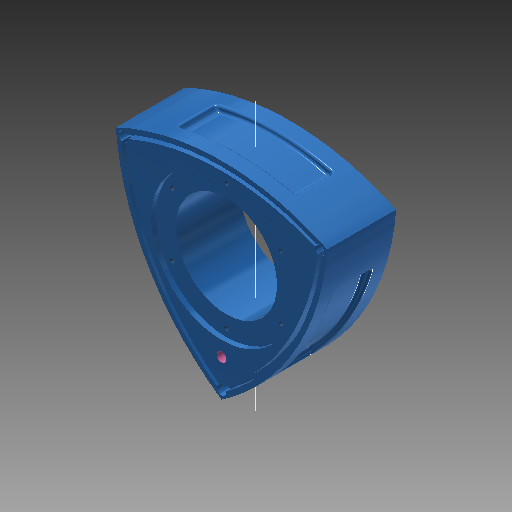
# Autodesk Inventor part: Rotor
Saved by Autodesk Inventor 2019.4 (Build 234330000, 330)
## iProperties
Created: 2020-05-01
Part Number: Rotor
Document SubType Name: Modeling
Designer: Gabriel
Material: Generic
Density: 1 g/cm^3
Appearance: Cyan
Author: Gabriel
Autodesk Inventor part; units mm, degrees
ref_plane "YZ Plane" through (0, 0, 0) normal (1, 0, 0) x (0, 1, 0)
ref_plane "XZ Plane" through (0, 0, 0) normal (0, 1, 0) x (-1, 0, 0)
sketch "Sketch1" plane through (0, 0, 0) normal (0, 0, 1) x (1, 0, 0)
  line L0 (0, 99.8581) -> (0, -123.3313) construction
  line L1 (-103.654, 0) -> (105.806, 0) construction
  line L2 (-287.8704, 0) -> (199.6451, 0) construction
  line L3 (0, -182) -> (0, 182) construction
  arc A0 (85.7365, 49.5) -> (-85.7365, 49.5) centre (0, -130) ccw
  arc A1 (-85.7365, 49.5) -> (0, -99) centre (112.5833, 65) ccw
  arc A2 (0, -99) -> (85.7365, 49.5) centre (-112.5833, 65) ccw
  circle A3 centre (0, 0) radius 41
  circle A4 centre (0, 0) radius 130 construction
  line L4 (0, 0) -> (-218.2253, 125.9925) construction
  circle A5 centre (0, 0) radius 99 construction
  dimension "d29" = 198
  dimension "d0" = 0
  dimension "d1" = 0
  dimension "d7" = 130
  dimension "d9" = 82
  dimension "d10" = 30
  constraints: 9 point on circle, 6 end point, 6 point on line, 5 centre point, 2 coincident, 2 equal radius, 1 midpoint, 1 perpendicular, 1 vertical, 3 other
  measures "d0" distance between parallel lines of L2 L1
  measures "d1" distance between parallel lines of L0 L3
  measures "d7" distance from line of L1 A0.centre
  measures "d9" diameter of A3
  measures "d10" angle of L1 L4
extrude "Extrusion1" add sketch "Sketch1" along normal mid plane 56
ref_plane "Work Plane1" through (0, -10, 0) normal (1, 0, 0) x (0, 1, 0)
sketch "Sketch3" plane through (0, 0, 28) normal (0, 0, 1) x (1, 0, 0)
  circle A0 centre (0, 0) radius 41 projected
  circle A1 centre (0, 0) radius 57
  dimension "d26" = 114
  constraints: 1 centre point, 1 coincident
  measures "d26" diameter of A1
extrude "Extrusion3" cut sketch "Sketch3" against normal blind 4
sketch "Sketch4" plane through (0, 0, 28) normal (0, 0, 1) x (1, 0, 0)
  circle A0 centre (0, 0) radius 57 projected
  arc A1 (85.7365, 49.5) -> (-85.7365, 49.5) centre (0, -130) ccw projected
  circle A2 centre (0, 0) radius 68.9246 construction
  circle A3 centre (0, -68.9246) radius 4
  circle A4 centre (0, 0) radius 41 projected
  line L0 (0, -169.8674) -> (0, 109.2044) projected
  line L1 (-120.6373, 0) -> (120.6373, 0) projected
  dimension "d30" = 8
  dimension "d32" = 0
  constraints: 1 centre point, 1 coincident, 1 vertical alignment, 3 other
  measures "d30" diameter of A3
  measures "d32" horizontal distance of A0.centre A3.centre
extrude "Extrusion4" cut sketch "Sketch4" against normal blind 10 contours A3 L0 | L0 A3
sketch "Sketch5" plane through (0, 0, 0) normal (0, 0, 1) x (1, 0, 0)
  line L0 (0, 126.8609) -> (0, -155.3102) projected
  line L1 (-71.353, 0) -> (71.353, 0) projected
  arc A0 (41.8711, 59.4241) -> (0, 65) centre (0, -95) ccw
  arc A1 (47.6756, 62.0624) -> (49.5197, 78.7726) centre (25.1952, 73) ccw
  arc A2 (49.5197, 78.7726) -> (0, 85) centre (0, -115) ccw
  arc A3 (41.8711, 59.4241) -> (47.6756, 62.0624) centre (43.1795, 64.2499) ccw
  arc A4 (0, 65) -> (-41.8711, 59.4241) centre (0, -95) ccw
  arc A5 (-49.5197, 78.7726) -> (-47.6756, 62.0624) centre (-25.1952, 73) ccw
  arc A6 (0, 85) -> (-49.5197, 78.7726) centre (0, -115) ccw
  arc A7 (-47.6756, 62.0624) -> (-41.8711, 59.4241) centre (-43.1795, 64.2499) ccw
  point P0 (0, 0)
  dimension "d35" = 160
  dimension "d36" = 95
  dimension "d37" = 200
  dimension "d38" = 115
  dimension "d39" = 25
  dimension "d40" = 73
  dimension "d41" = 5
  constraints: 18 point on circle, 8 centre point, 5 symmetric about line, 4 point on line, 2 tangent, 4 other
  measures "d35" radius of A0
  measures "d36" distance of A0.centre point (0, 0)
  measures "d37" radius of A2
  measures "d38" distance of A2.centre point (0, 0)
  measures "d39" radius of A1
  measures "d40" distance from line of L1 A1.centre
  measures "d41" radius of A3
extrude "Extrusion5" cut sketch "Sketch5" along normal mid plane 30
fillet "Fillet1" radius 2 10 edges at (45.2484, 59.698, 15) (47.9008, 62.5378, 15) (-45.2484, 59.698, 15) (-47.9008, 62.5378, 15) (0, 65, 15) (-45.2484, 59.698, -15) (-47.9008, 62.5378, -15) (45.2484, 59.698, -15) (47.9008, 62.5378, -15) (0, 65, -15)
fillet "Fillet2" radius 2 8 edges at (47.6308, 63.138, 14.3144) (0, 68.9246, 15) (-47.6308, 63.138, 14.3144) (-48.1159, 63.0178, 0) (-47.6308, 63.138, -14.3144) (0, 68.9246, -15) (47.6308, 63.138, -14.3144) (48.1159, 63.0178, 0)
pattern_circular "Circular Pattern1" count 3 over 360 about axis through (0, 0, 0) along (0, 0, 1) of "Extrusion5"
pattern_circular "Circular Pattern2" count 3 over 360 about axis through (0, 0, 0) along (0, 0, 1) of "Fillet1", "Fillet2"
sketch "Sketch7" plane through (0, 0, 24) normal (0, 0, 1) x (1, 0, 0)
  line L0 (0, 102.5095) -> (0, -132.5849) projected
  line L1 (-120.0311, 0) -> (120.0311, 0) projected
  point P0 (0, 51)
  dimension "d60" = 51
  constraints: 1 point on line
  measures "d60" distance from line of L1 point (0, 51)
hole "Hole3" at (0, 51, 24) direction (0, 0, -1) diameter 3.242 depth 11.8 tip angle 118 thread size "M4x0.7" class "6H" standard "ISO Metric profile"
pattern_circular "Circular Pattern3" count 6 over 360 about axis through (0, 0, 0) along (0, 0, 1) of "Hole3"
sketch "Sketch8" plane through (0, 0, 28) normal (0, 0, 1) x (1, 0, 0)
  arc A0 (-85.7365, 49.5) -> (0, -99) centre (112.5833, 65) ccw projected
  arc A1 (85.7365, 49.5) -> (-85.7365, 49.5) centre (0, -130) ccw projected
  arc A2 (0, -99) -> (85.7365, 49.5) centre (-112.5833, 65) ccw projected
  arc A3 (81.5142, 47.0622) -> (-81.5142, 47.0622) centre (0, -130) ccw
  arc A4 (-81.5142, 47.0622) -> (0, -94.1245) centre (112.5833, 65) ccw
  arc A5 (0, -94.1245) -> (81.5142, 47.0622) centre (-112.5833, 65) ccw
  arc A6 (78.3191, 45.2175) -> (-78.3191, 45.2175) centre (0, -130) ccw
  arc A7 (-78.3191, 45.2175) -> (0, -90.4351) centre (112.5833, 65) ccw
  arc A8 (0, -90.4351) -> (78.3191, 45.2175) centre (-112.5833, 65) ccw
  dimension "d71" = 4
  dimension "d72" = 3
  constraints: 12 point on circle, 6 centre point, 4 other
  measures "d71" radial gap between concentric circles of A2 A5
  measures "d72" radial gap between concentric circles of A5 A8
extrude "Extrusion6" cut sketch "Sketch8" against normal blind 7 contours A5 A4 A3
sketch "Sketch9" plane through (0, 0, 28) normal (0, 0, 1) x (1, 0, 0)
  arc A0 (85.7365, 49.5) -> (-85.7365, 49.5) centre (0, -130) ccw projected
  arc A1 (-85.7365, 49.5) -> (0, -99) centre (112.5833, 65) ccw projected
  arc A2 (0, -99) -> (85.7365, 49.5) centre (-112.5833, 65) ccw projected
  arc A3 (-81.5142, 47.0622) -> (0, -94.1245) centre (112.5833, 65) ccw projected
  arc A4 (81.5142, 47.0622) -> (-81.5142, 47.0622) centre (0, -130) ccw projected
  arc A5 (0, -94.1245) -> (81.5142, 47.0622) centre (-112.5833, 65) ccw projected
  point P0 (0, -92)
  point P1 (79.6743, 46)
  point P2 (-79.6743, 46)
  dimension "d75" = 7
  dimension "d76" = 0
  dimension "d77" = 6.0622
  dimension "d78" = 3.5
  dimension "d79" = 6.0622
  constraints: 1 horizontal alignment
  measures "d75" distance of point (0, -92) A1.end
  measures "d76" horizontal distance of point (0, -92) A3.end
  measures "d77" horizontal distance of point (79.674, 46) A0.start
  measures "d78" vertical distance of A0.start point (79.674, 46)
  measures "d79" horizontal distance of A0.end point (-79.674, 46)
hole "Hole4" at (0, -92, 28) at (79.6743, 46, 28) at (-79.6743, 46, 28) direction (0, 0, -1) diameter 8 depth 8
mirror "Mirror1" about plane through (0, 0, 0) normal (0, 0, 1) of "Extrusion6", "Hole4"
sketch "Sketch10" plane through (0, 0, -28) normal (0, 0, -1) x (-1, 0, 0)
  arc A0 (62.9274, 9.7551) -> (69.5295, 38.7143) centre (-112.5833, 65) ccw
  arc A1 (68.2923, 40.8571) -> (39.9119, 49.6192) centre (0, -130) ccw
  arc A2 (59.0479, 10.021) -> (38.2024, 46.1265) centre (0, 0) ccw
  arc A3 (0, -99) -> (85.7365, 49.5) centre (-112.5833, 65) ccw projected
  arc A4 (85.7365, 49.5) -> (-85.7365, 49.5) centre (0, -130) ccw projected
  circle A5 centre (0, 0) radius 41 projected
  arc A6 (59.0479, 10.021) -> (62.9274, 9.7551) centre (61.0197, 10.3556) ccw
  arc A7 (39.9119, 49.6192) -> (38.2024, 46.1265) centre (39.4781, 47.6668) ccw
  arc A8 (69.5295, 38.7143) -> (68.2923, 40.8571) centre (67.55, 39) ccw
  dimension "d87" = 184
  dimension "d88" = 184
  dimension "d89" = 59.8922
  dimension "d90" = 2
  constraints: 12 point on circle, 6 centre point, 6 tangent, 3 concentric, 2 equal radius
  measures "d87" radius of A0
  measures "d88" radius of A1
  measures "d89" radius of A2
  measures "d90" radius of A6
extrude "Extrusion7" cut sketch "Sketch10" against normal blind 30 contours A6 A2 A7 A1 A8 A0
pattern_circular "Circular Pattern4" count 3 over 360 about axis through (0, 0, 0) along (0, 0, 1) of "Extrusion7"
sketch "Sketch11" plane through (0, 0, -28) normal (0, 0, -1) x (-1, 0, 0)
  arc A0 (31.0444, -47.8042) -> (56.7831, -4.9679) centre (0, 0) ccw
  arc A1 (26.6873, -41.0949) -> (48.8135, -4.2706) centre (0, 0) ccw
  circle A2 centre (0, 0) radius 41 projected
  arc A3 (26.6873, -41.0949) -> (31.0444, -47.8042) centre (28.8659, -44.4495) ccw
  arc A4 (56.7831, -4.9679) -> (48.8135, -4.2706) centre (52.7983, -4.6193) ccw
  line L0 (0, 0) -> (28.8659, -44.4495) construction
  line L1 (0, 0) -> (52.7983, -4.6193) construction
  line L2 (-120.0311, 0) -> (120.0311, 0) construction
  dimension "d96" = 57
  dimension "d97" = 49
  dimension "d98" = 5
  dimension "d99" = 52
  constraints: 8 point on circle, 4 centre point, 4 end point, 4 tangent, 2 concentric
  measures "d96" radius of A0
  measures "d97" radius of A1
  measures "d98" angle of L2 L1
  measures "d99" angle of L0 L1
extrude "Extrusion8" cut sketch "Sketch11" against normal blind 30 contours A3 A1 A4 A0
pattern_circular "Circular Pattern5" count 3 over 360 about axis through (0, 0, 0) along (0, 0, 1) of "Extrusion8"
equation "\"d79\" = d77"
equation "\"d88\" = d87"
equation "\"d100\" = d91"
equation "\"d91\" = 30"
body "Solid1"
